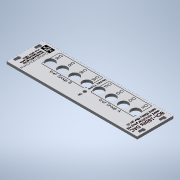
# Autodesk Inventor part: Frontplate_Dac8728_v12_decal
Saved by Autodesk Inventor 2022 (Build 260153000, 153)
## iProperties
Created: 2022-10-26
Part Number: Frontplate_Dac8728_v12_decal
Material: Generic
Document SubType Name: Modeling
Designer: Baaij
Density: 1 g/cm^3
Appearance: Default
Author: Baaij
Autodesk Inventor part; units mm, degrees
ref_plane "YZ Plane" through (0, 0, 0) normal (1, 0, 0) x (0, 1, 0)
ref_plane "XZ Plane" through (0, 0, 0) normal (0, 1, 0) x (-1, 0, 0)
sketch "Sketch1" plane through (0, 0, 0) normal (0, 0, 1) x (1, 0, 0)
  line L0 (-64.2, 21.11) -> (64.2, 21.11)
  line L1 (64.2, 21.11) -> (64.2, -14.25)
  line L2 (64.2, -14.25) -> (-64.2, -14.25)
  line L3 (-64.2, -14.25) -> (-64.2, 21.11)
  line L4 (-59.65, 16.1384) -> (-59.65, 11.1816)
  line L5 (-62.85, 11.1816) -> (-62.85, 16.1384)
  line L6 (-64.2, 0) -> (64.2, 0) construction
  line L7 (-62.85, 16.1384) -> (-62.85, 11.1816)
  line L8 (-59.65, 16.1384) -> (-59.65, 11.1816)
  arc A0 (-59.65, 16.1384) -> (-62.85, 16.1384) centre (-61.25, 13.66) ccw
  arc A1 (-62.85, 11.1816) -> (-59.65, 11.1816) centre (-61.25, 13.66) ccw
  line L9 (-50, -1.6) -> (50, -1.6) construction
  line L10 (64.2, -11.9) -> (-64.2, -11.9) construction
  line L11 (0, 28.2591) -> (0, -21.7844) construction
  line L12 (-94.5, 0) -> (94.5, 0) construction
  line L13 (67.5, 3.43) -> (-67.5, 3.43) construction
  line L14 (50, 0) -> (50, -1.6) construction
  line L15 (-50, 0) -> (-50, -1.6) construction
  point P0 (0, 0)
  point P1 (-34.25, -9.4)
  point P2 (-42, 6.4)
  point P3 (0, -1.6)
  dimension "d0" = 128.4
  dimension "d1" = 35.36
  dimension "d21" = 6.4
  dimension "d46" = 1.6
  dimension "d47" = 1.6
  dimension "d50" = 2.95
  dimension "d52" = 2.95
  dimension "d130" = 2.35
  dimension "d131" = 11.9
  dimension "d132" = 10.3
  dimension "d133" = 2.5
  dimension "d145" = 0
  dimension "d152" = 135
  dimension "d155" = 17.68
  dimension "d156" = 10.23
  dimension "d157" = 64.2
  dimension "d158" = 61.25
  dimension "d159" = 67.5
  dimension "d215" = 50
  dimension "d217" = 50
  dimension "d218" = 8
  dimension "d219" = 0
  dimension "d227" = 34.25
  constraints: 28 end point, 8 perpendicular, 7 point on line, 4 point on circle, 3 horizontal, 3 parallel, 2 centre point, 1 coincident, 1 vertical
  measures "d0" distance of L1.end L2.end
  measures "d1" distance of L0.end L1.end
  measures "d21" distance from line of L6 point (-42, 6.4)
  measures "d46" distance from line of L8 A0.centre
  measures "d47" distance from line of L5 A0.centre
  measures "d50" radius of A0
  measures "d52" radius of A1
  measures "d130" distance between parallel lines of L2 L10
  measures "d131" distance between parallel lines of L10 L6
  measures "d132" distance between parallel lines of L10 L9
  measures "d133" distance from line of L10 point (-34.25, -9.4)
  measures "d145" distance from line of L6 point (0, 0)
  measures "d152" distance of L13.end L13.start
  measures "d155" distance between parallel lines of L13 L0
  measures "d156" distance from line of L13 A0.centre
  measures "d157" distance between parallel lines of L11 L3
  measures "d158" distance from line of L11 A0.centre
  measures "d159" distance from line of L11 L13.start
  measures "d215" distance from line of L9.end L11
  measures "d217" distance between parallel lines of L11 L15
  measures "d218" horizontal distance of L15.start point (-42, 6.4)
  measures "d219" distance from line of point (0, -1.6) L9
  measures "d227" distance from line of point (-34.25, -9.4) L11
extrude "Extrusion2" add sketch "Sketch1" along normal blind 2.5 contours L0 L1 L2 L3 | L4 A1 L5 A0
hole "Hole1" at (-42, 6.4, 0) direction (0, 0, 1) diameter 9 end through all
pattern_linear "Rectangular Pattern1" count 8 spacing 12 along (1, 0, 0) of "Hole1"
extrude "Extrusion3" cut sketch "Sketch1" along normal blind 2.5 contours L4 A1 L5 A0
pattern_linear "Rectangular Pattern2" count 2 spacing 122.5 along (1, 0, 0) count 2 spacing -20.46 along (0, 1, 0) of "Extrusion3"
hole "Hole9" at (-61.25, 13.66, 0) at (0, -1.6, 0) direction (0, 0, 1) diameter 3.2 end through all
ref_plane "Work Plane1" through (0, 0, 2.5) normal (0, 0, 1) x (1, 0, 0)
sketch "Sketch7" plane through (0, 0, 2.5) normal (0, 0, 1) x (1, 0, 0)
  line L0 (64.2, -14.25) -> (64.2, 21.11) projected
  line L1 (64.2, 21.11) -> (64.2, -14.501) construction
  line L2 (64.2, -14.501) -> (-64.2197, -14.501) construction
  line L3 (-64.2197, -14.501) -> (-64.2197, 21.11) construction
  line L4 (-64.2197, 21.11) -> (64.2, 21.11) construction
  point P0 (0, 0)
  constraints: 2 other
decal "Decal4"
body "Solid2"
